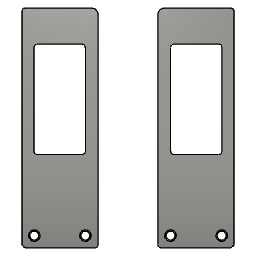
mriya-cnc-display-cover (Autodesk Fusion 360 design; units mm, degrees)
Autodesk Fusion 360 part; units mm, degrees
note: some values were not read from the file. Set by a fixed rule: which sketch regions a step uses.
sketch "mriya-display-cover" plane through (0, 0, 0) normal (0, 0, 1) x (1, 0, 0)
  circle A0 centre (-22.9, 19.5) radius 1.1
  circle A1 centre (-10.4, 19.5) radius 1.1
  circle A2 centre (-22.9, 19.5) radius 1.4
  circle A3 centre (-10.4, 19.5) radius 1.4
  line L0 (-23.7, 36.2) -> (-23.7, 71.8)
  line L1 (-10.5, 35.4) -> (-22.9, 35.4)
  line L2 (-11.25, 39.3) -> (-22.15, 39.3)
  arc A4 (-10.5, 35.4) -> (-9.7, 36.2) centre (-10.5, 36.2) ccw
  arc A5 (-22.9, 72.6) -> (-23.7, 71.8) centre (-22.9, 71.8) ccw
  line L3 (-22.15, 66.3) -> (-11.25, 66.3)
  line L4 (-10.5, 72.6) -> (-22.9, 72.6)
  line L5 (-22.95, 65.5) -> (-22.95, 40.1)
  arc A6 (-9.7, 71.8) -> (-10.5, 72.6) centre (-10.5, 71.8) ccw
  arc A7 (-23.7, 36.2) -> (-22.9, 35.4) centre (-22.9, 36.2) ccw
  line L6 (-10.45, 40.1) -> (-10.45, 65.5)
  line L7 (-9.7, 71.8) -> (-9.7, 36.2)
  arc A8 (-22.95, 40.1) -> (-22.15, 39.3) centre (-22.15, 40.1) ccw
  arc A9 (-11.25, 39.3) -> (-10.45, 40.1) centre (-11.25, 40.1) ccw
  arc A10 (-22.15, 66.3) -> (-22.95, 65.5) centre (-22.15, 65.5) ccw
  arc A11 (-10.45, 65.5) -> (-11.25, 66.3) centre (-11.25, 65.5) ccw
  line L8 (-25.9, 17.5) -> (-25.9, 74.3)
  line L9 (-8.9, 75.1) -> (-25.1, 75.1)
  line L10 (-7.3, 73.5) -> (-7.3, 17.3)
  arc A12 (-8.1, 16.5) -> (-7.3, 17.3) centre (-8.1, 17.3) ccw
  arc A13 (-25.1, 75.1) -> (-25.9, 74.3) centre (-25.1, 74.3) ccw
  line L11 (-24.9, 16.5) -> (-8.1, 16.5)
  arc A14 (-7.3, 73.5) -> (-8.9, 75.1) centre (-8.9, 73.5) ccw
  arc A15 (-25.9, 17.5) -> (-24.9, 16.5) centre (-24.9, 17.5) ccw
  point P0 (-23.7, 35.4)
  point P1 (-23.7, 72.6)
  point P2 (-8.8, 35)
  point P3 (-9.7, 35.4)
  point P4 (-9.7, 72.6)
  point P5 (-8.8, 32.8)
  dimension "d8" = 2.2
  dimension "d9" = 2.2
  dimension "d17" = 2.8
  dimension "d18" = 2.8
  constraint concentric A1 A3
  constraint perpendicular L1 L7
  constraint perpendicular L2 L5
  constraint coincident P4 L7
  constraint tangent A6 L7
  constraint coincident P1 L0
  constraint tangent L0 A5
  constraint coincident P3 L1
  constraint coincident P3 L7
  constraint tangent L1 A4
  constraint tangent A4 L7
  constraint coincident P0 L0
  constraint coincident P0 L1
  constraint tangent L0 A7
  constraint tangent L1 A7
  constraint tangent A5 L4
  constraint vertical L5
  constraint perpendicular L3 L5
  constraint vertical L6
  constraint tangent L5 A8
  constraint tangent L2 A8
  constraint tangent L6 A9
  constraint tangent L2 A9
  constraint tangent L3 A10
  constraint tangent L5 A10
  constraint tangent L3 A11
  constraint tangent L6 A11
  constraint perpendicular L8 L9
  constraint tangent L10 A12
  constraint tangent L8 A13
  constraint tangent L9 A13
  constraint tangent A12 L11
  constraint tangent L10 A14
  constraint tangent L9 A14
  constraint horizontal L11
  constraint perpendicular L8 L11
  constraint tangent L8 A15
  constraint tangent L11 A15
  measures "d8" diameter of A0
  measures "d9" diameter of A1
  measures "d17" diameter of A2
  measures "d18" diameter of A3
extrude "Extrude5" add sketch "mriya-display-cover" along normal blind 1.5 contours L8 L9 L10 A12 A13 L11 A14 A15 makes body 1
extrude "Extrude6" add sketch "mriya-display-cover" along normal blind 0.7 contours A2 | A3 bodies 1
extrude "Extrude7" add sketch "mriya-display-cover" along normal blind 0.5 from surface at 1 contours L0 L1 A4 A5 L4 A6 A7 L7 bodies 1
mirror "Mirror2" about plane through (0, 0, 0) normal (1, 0, 0) of bodies 1 makes body 2
named bodies: "Left", "Right"
